Autodesk Inventor part; units mm, degrees
(part 4 of 4)
sketch "Эскиз25" plane through (0, 0, 5) normal (0, 0, 1) x (1, 0, 0)
  circle A0 centre (1.2104, 5.1192) radius 2.5 projected
  circle A1 centre (4.7663, 12.2855) radius 1.6 projected
  circle A2 centre (-5.9559, 8.675) radius 1.6 projected
  circle A3 centre (-2.3455, -2.0471) radius 1.6 projected
  circle A4 centre (8.3767, 1.5633) radius 1.6 projected
  line L0 (-21.1743, 35.425) -> (-40.4462, 33.5769) projected
  line L1 (-40.4462, 33.5769) -> (-39.7656, 26.479) projected
  line L2 (-39.7656, 26.479) -> (-20.2818, 28.3476) projected
  line L3 (-20.2818, 28.3476) -> (-17.326, 27.8341) projected
  line L4 (-17.326, 27.8341) -> (-9.2052, 11.8155) projected
  arc A5 (-9.2052, 11.8155) -> (-10.7875, 8.1814) centre (1.2104, 5.1192) ccw projected
  arc A6 (-10.7875, 8.1814) -> (-13.7875, 7.8251) centre (-10.997, -2.8603) ccw projected
  arc A7 (-13.7875, 7.8251) -> (-13.9423, 6.7483) centre (1.2104, 5.1192) ccw projected
  arc A8 (-13.9423, 6.7483) -> (-11.1642, 5.5611) centre (-8.2544, 16.2146) ccw projected
  arc A9 (-11.1642, 5.5611) -> (-11.1642, 4.6772) centre (1.2104, 5.1192) ccw projected
  arc A10 (-11.1642, 4.6772) -> (-13.9423, 3.4901) centre (-8.2544, -5.9763) ccw projected
  arc A11 (-13.9423, 3.4901) -> (-13.7875, 2.4133) centre (1.2104, 5.1192) ccw projected
  arc A12 (-13.7875, 2.4133) -> (-10.7875, 2.0569) centre (-10.997, 13.0986) ccw projected
  arc A13 (-10.7875, 2.0569) -> (-10.5384, 1.2088) centre (1.2104, 5.1192) ccw projected
  arc A14 (-10.5384, 1.2088) -> (-12.8695, -0.7129) centre (-4.7451, -8.1934) ccw projected
  arc A15 (-12.8695, -0.7129) -> (-12.4176, -1.7025) centre (1.2104, 5.1192) ccw projected
  arc A16 (-12.4176, -1.7025) -> (-9.4387, -1.1992) centre (-12.7506, 9.3362) ccw projected
  arc A17 (-9.4387, -1.1992) -> (-8.9608, -1.9429) centre (1.2104, 5.1192) ccw projected
  arc A18 (-8.9608, -1.9429) -> (-10.6561, -4.4435) centre (-0.7533, -9.332) ccw projected
  arc A19 (-10.6561, -4.4435) -> (-9.9437, -5.2656) centre (1.2104, 5.1192) ccw projected
  arc A20 (-9.9437, -5.2656) -> (-7.2273, -3.9435) centre (-13.3732, 5.2321) ccw projected
  arc A21 (-7.2273, -3.9435) -> (-6.5592, -4.5224) centre (1.2104, 5.1192) ccw projected
  arc A22 (-6.5592, -4.5224) -> (-7.4813, -7.3993) centre (3.3977, -9.2999) ccw projected
  arc A23 (-7.4813, -7.3993) -> (-6.5661, -7.9874) centre (1.2104, 5.1192) ccw projected
  arc A24 (-6.5661, -7.9874) -> (-4.3322, -5.9536) centre (-12.8142, 1.1189) ccw projected
  arc A25 (-4.3322, -5.9536) -> (-3.5282, -6.3208) centre (1.2104, 5.1192) ccw projected
  arc A26 (-3.5282, -6.3208) -> (-3.6024, -9.3409) centre (7.3714, -8.0996) ccw projected
  arc A27 (-3.6024, -9.3409) -> (-2.5586, -9.6474) centre (1.2104, 5.1192) ccw projected
  arc A28 (-2.5586, -9.6474) -> (-0.9882, -7.0666) centre (-11.1191, -2.6703) ccw projected
  arc A29 (-0.9882, -7.0666) -> (-0.1132, -7.1924) centre (1.2104, 5.1192) ccw projected
  arc A30 (-0.1132, -7.1924) -> (0.6664, -10.1111) centre (10.846, -5.8284) ccw projected
  arc A31 (0.6664, -10.1111) -> (1.7543, -10.1111) centre (1.2104, 5.1192) ccw projected
  arc A32 (1.7543, -10.1111) -> (2.534, -7.1924) centre (-8.4252, -5.8284) ccw projected
  arc A33 (2.534, -7.1924) -> (3.409, -7.0666) centre (1.2104, 5.1192) ccw projected
  arc A34 (3.409, -7.0666) -> (4.9793, -9.6474) centre (13.5399, -2.6703) ccw projected
  arc A35 (4.9793, -9.6474) -> (6.0232, -9.3409) centre (1.2104, 5.1192) ccw projected
  arc A36 (6.0232, -9.3409) -> (5.949, -6.3208) centre (-4.9506, -8.0996) ccw projected
  arc A37 (5.949, -6.3208) -> (6.7442, -5.958) centre (1.2104, 5.1192) ccw projected
  arc A38 (6.7442, -5.958) -> (8.9765, -7.9936) centre (15.2319, 1.1078) ccw projected
  arc A39 (8.9765, -7.9936) -> (9.8922, -7.4062) centre (1.2104, 5.1192) ccw projected
  arc A40 (9.8922, -7.4062) -> (8.9724, -4.5285) centre (-0.9883, -9.2981) ccw projected
  arc A41 (8.9724, -4.5285) -> (9.6409, -3.9502) centre (1.2104, 5.1192) ccw projected
  arc A42 (9.6409, -3.9502) -> (12.3562, -5.2745) centre (15.794, 5.2205) ccw projected
  arc A43 (12.3562, -5.2745) -> (13.0693, -4.4529) centre (1.2104, 5.1192) ccw projected
  arc A44 (13.0693, -4.4529) -> (11.376, -1.9509) centre (3.1626, -9.3336) ccw projected
  arc A45 (11.376, -1.9509) -> (11.8545, -1.2077) centre (1.2104, 5.1192) ccw projected
  arc A46 (11.8545, -1.2077) -> (14.833, -1.7133) centre (15.1747, 9.3251) ccw projected
  arc A47 (14.833, -1.7133) -> (15.2857, -0.7241) centre (1.2104, 5.1192) ccw projected
  arc A48 (15.2857, -0.7241) -> (12.9561, 1.1995) centre (7.1553, -8.1981) ccw projected
  arc A49 (12.9561, 1.1995) -> (8.4894, 15.1363) centre (1.2104, 5.1192) ccw projected
  line L5 (8.4894, 15.1363) -> (-17.35, 43.8487) projected
  line L6 (-17.35, 43.8487) -> (-22.1564, 44.6837) projected
  line L7 (-22.1564, 44.6837) -> (-44.9679, 42.4962) projected
  line L8 (-44.9679, 42.4962) -> (-44.2873, 35.3983) projected
  line L9 (-44.2873, 35.3983) -> (-24.8035, 37.2669) projected
  line L10 (-24.8035, 37.2669) -> (-21.8477, 36.7534) projected
  line L11 (-21.8477, 36.7534) -> (-21.1743, 35.425) projected
  line L12 (-17.326, 27.8341) -> (-37.8384, 68.2957)
  point P0 (0, 0)
  constraints: 2 end point, 1 collinear
extrude "Выдавливание23" cut sketch "Эскиз25" against normal through all contours L12 L3 L2 L1 L0
